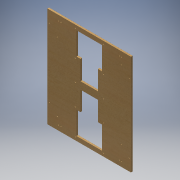
# Autodesk Inventor part: socle-robot
Saved by Autodesk Inventor 2019 (Build 230136000, 136)
## iProperties
Created: 2018-04-01
Part Number: socle-robot
Material: Generic
Document SubType Name: Modeling
Designer: franc
Density: 1 g/cm^3
Appearance: Pin jaune - Massif moiré clair faible lustre
Mass: 292.807 g
Surface Area: 1271.34 cm^2
Volume: 292.807 cm^3
Author: franc
Autodesk Inventor part; units mm, degrees
ref_plane "YZ Plane" through (0, 0, 0) normal (1, 0, 0) x (0, 1, 0)
ref_plane "XZ Plane" through (0, 0, 0) normal (0, 1, 0) x (-1, 0, 0)
ref_plane "XY Plane" through (0, 0, 0) normal (0, 0, 1) x (1, 0, 0)
sketch "Esquisse1" plane through (0, 0, 0) normal (0, 1, 0) x (-1, 0, 0)
  line L0 (81.9588, 98.0854) -> (-168.0412, 98.0854)
  line L1 (-168.0412, 98.0854) -> (-168.0412, -201.9146)
  line L2 (-168.0412, -201.9146) -> (81.9588, -201.9146)
  line L3 (81.9588, -201.9146) -> (81.9588, 98.0854)
  point P0 (0, 0)
  dimension "d0" = 300
  dimension "d1" = 250
  constraints: 8 end point, 2 parallel, 1 horizontal, 1 perpendicular
  measures "d0" distance of L2.end L0.start
  measures "d1" distance of L0.start L0.end
extrude "Extrusion1" add sketch "Esquisse1" along normal blind 5
sketch "Sketch3" plane through (0, 5, 0) normal (0, 1, 0) x (1, 0, 0)
  line L0 (81.0412, -85.0854) -> (5.0412, -85.0854)
  line L1 (5.0412, -85.0854) -> (5.0412, -17.0854)
  line L2 (81.0412, -17.0854) -> (81.0412, -85.0854)
  line L3 (-81.9588, -98.0854) -> (168.0412, -98.0854) projected
  line L4 (168.0412, -98.0854) -> (168.0412, 201.9146) projected
  line L5 (17.0412, -17.0854) -> (17.0412, 40.9146)
  line L6 (17.0412, 40.9146) -> (69.0412, 40.9146)
  line L7 (69.0412, 40.9146) -> (69.0412, -17.0854)
  line L8 (5.0412, -17.0854) -> (17.0412, -17.0854)
  line L9 (69.0412, -17.0854) -> (81.0412, -17.0854)
  line L10 (81.0412, 188.9146) -> (5.0412, 188.9146)
  line L11 (5.0412, 188.9146) -> (5.0412, 120.9146)
  line L12 (81.0412, 120.9146) -> (81.0412, 188.9146)
  line L13 (168.0412, 201.9146) -> (-81.9588, 201.9146) projected
  line L14 (17.0412, 120.9146) -> (17.0412, 62.9146)
  line L15 (17.0412, 62.9146) -> (69.0412, 62.9146)
  line L16 (69.0412, 62.9146) -> (69.0412, 120.9146)
  line L17 (5.0412, 120.9146) -> (17.0412, 120.9146)
  line L18 (69.0412, 120.9146) -> (81.0412, 120.9146)
  circle A0 centre (85.0412, 51.9146) radius 1.5
  line L19 (-81.9588, 201.9146) -> (-81.9588, -98.0854) projected
  circle A1 centre (1.0412, 51.9146) radius 1.5
  point P0 (0, 0)
  dimension "d17" = 76
  dimension "d18" = 68
  dimension "d19" = 13
  dimension "d20" = 87
  dimension "d21" = 12
  dimension "d22" = 12
  dimension "d23" = 58
  dimension "d24" = 68
  dimension "d25" = 52
  dimension "d26" = 13
  dimension "d27" = 76
  dimension "d28" = 68
  dimension "d29" = 87
  dimension "d30" = 12
  dimension "d31" = 12
  dimension "d32" = 58
  dimension "d33" = 52
  dimension "d34" = 68
  dimension "d39" = 3
  dimension "d53" = 83
  dimension "d54" = 150
  dimension "d58" = 3
  dimension "d59" = 83
  dimension "d60" = 150
  constraints: 32 end point, 8 parallel, 2 centre point, 2 horizontal, 2 perpendicular
  measures "d17" distance of L1.end L2.start
  measures "d18" distance of L0.end L1.end
  measures "d19" distance between parallel lines of L3 L0
  measures "d20" distance between parallel lines of L4 L2
  measures "d21" distance between parallel lines of L2 L7
  measures "d22" distance between parallel lines of L1 L5
  measures "d23" distance of L6.end L7.end
  measures "d24" distance of L2.start L0.start
  measures "d25" distance of L5.end L6.end
  measures "d26" distance between parallel lines of L13 L10
  measures "d27" distance of L10.start L10.end
  measures "d28" distance of L12.start L10.start
  measures "d29" distance between parallel lines of L4 L12
  measures "d30" distance between parallel lines of L12 L16
  measures "d31" distance between parallel lines of L11 L14
  measures "d32" distance of L15.end L16.end
  measures "d33" distance of L14.end L15.end
  measures "d34" distance of L10.end L11.end
  measures "d39" diameter of A0
  measures "d53" distance from line of L4 A0.centre
  measures "d54" distance from line of L3 A0.centre
  measures "d58" diameter of A1
  measures "d59" distance from line of L19 A1.centre
  measures "d60" distance from line of L3 A1.centre
extrude "Extrusion3" cut sketch "Sketch3" against normal through all contours L0 L1 L8 L5 L6 L7 L9 L2 | L12 L18 L16 L15 L14 L17 L11 L10 | A0 | A1
sketch "Sketch4" plane through (0, 5, 0) normal (0, 1, 0) x (1, 0, 0)
  circle A0 centre (1.0412, -89.0854) radius 1.5 projected
  circle A1 centre (1.0412, -11.0854) radius 1.5 projected
  circle A2 centre (85.0412, -89.0854) radius 1.5 projected
  circle A3 centre (85.0412, -11.0854) radius 1.5 projected
  circle A4 centre (1.0412, 114.9146) radius 1.5 projected
  circle A5 centre (1.0412, 192.9146) radius 1.5 projected
  circle A6 centre (85.0412, 192.9146) radius 1.5 projected
  circle A7 centre (85.0412, 114.9146) radius 1.5 projected
  point P0 (0, 0)
extrude "Extrusion4" cut sketch "Sketch4" against normal up to next
sketch "Esquisse5" plane through (0, 5, 0) normal (0, 1, 0) x (1, 0, 0)
  circle A0 centre (139.5412, -83.0854) radius 1.5 projected
  circle A1 centre (133.0412, -83.0854) radius 1.5 projected
  circle A2 centre (133.0412, 186.9146) radius 1.5 projected
  circle A3 centre (139.5412, 186.9146) radius 1.5 projected
  circle A4 centre (-41.9588, 186.9146) radius 1.5 projected
  circle A5 centre (-48.4588, 186.9145) radius 1.4999 projected
  circle A6 centre (-41.9588, -83.0854) radius 1.5 projected
  circle A7 centre (85.0412, 192.9146) radius 1.5 projected
  circle A8 centre (1.0412, 114.9146) radius 1.5 projected
  circle A9 centre (85.0412, -89.0854) radius 1.5 projected
  circle A10 centre (1.0412, -89.0854) radius 1.5 projected
  circle A11 centre (1.0412, -11.0854) radius 1.5 projected
  circle A12 centre (85.0412, -11.0854) radius 1.5 projected
  circle A13 centre (1.0412, 192.9146) radius 1.5 projected
  circle A14 centre (85.0412, 114.9146) radius 1.5 projected
  line L0 (81.0412, -17.0854) -> (81.0412, -85.0854) projected
  line L1 (81.0412, -85.0854) -> (5.0412, -85.0854) projected
  line L2 (5.0412, -85.0854) -> (5.0412, -17.0854) projected
  line L3 (5.0412, -17.0854) -> (17.0412, -17.0854) projected
  line L4 (17.0412, -17.0854) -> (17.0412, 40.9146) projected
  line L5 (17.0412, 40.9146) -> (69.0412, 40.9146) projected
  line L6 (69.0412, 40.9146) -> (69.0412, -17.0854) projected
  line L7 (69.0412, -17.0854) -> (81.0412, -17.0854) projected
  circle A15 centre (85.0412, 51.9146) radius 1.5 projected
  circle A16 centre (1.0412, 51.9146) radius 1.5 projected
  line L8 (5.0412, 120.9146) -> (5.0412, 188.9146) projected
  line L9 (5.0412, 188.9146) -> (81.0412, 188.9146) projected
  line L10 (81.0412, 188.9146) -> (81.0412, 120.9146) projected
  line L11 (81.0412, 120.9146) -> (69.0412, 120.9146) projected
  line L12 (69.0412, 120.9146) -> (69.0412, 62.9146) projected
  line L13 (69.0412, 62.9146) -> (17.0412, 62.9146) projected
  line L14 (17.0412, 62.9146) -> (17.0412, 120.9146) projected
  line L15 (17.0412, 120.9146) -> (5.0412, 120.9146) projected
  line L16 (-81.9588, -98.0854) -> (168.0412, -98.0854) projected
  line L17 (168.0412, -98.0854) -> (168.0412, 201.9146) projected
  line L18 (168.0412, 201.9146) -> (-81.9588, 201.9146) projected
  line L19 (-81.9588, 201.9146) -> (-81.9588, -98.0854) projected
  circle A17 centre (-48.4588, -83.0854) radius 1.5 projected
  point P0 (0, 0)
extrude "Extrusion5" cut sketch "Esquisse5" against normal up to next contours A0 | A1 | A2 | A3 | A4 | A5 | A6 | A17
sketch "Esquisse6" plane through (0, 0, 0) normal (0, -1, 0) x (1, 0, 0)
  circle A0 centre (-76.9588, -142.9146) radius 1.5 projected
  circle A1 centre (-52.9588, -166.9146) radius 1.5 projected
  circle A2 centre (-76.9588, 63.0854) radius 1.5 projected
  circle A3 centre (-52.9588, 39.0854) radius 1.5 projected
  circle A4 centre (139.0412, 63.0854) radius 1.5 projected
  circle A5 centre (163.0412, 39.0854) radius 1.5 projected
  circle A6 centre (139.0412, -142.9146) radius 1.5 projected
  circle A7 centre (163.0412, -166.9146) radius 1.5 projected
  point P0 (0, 0)
extrude "Extrusion6" cut sketch "Esquisse6" against normal up to next
